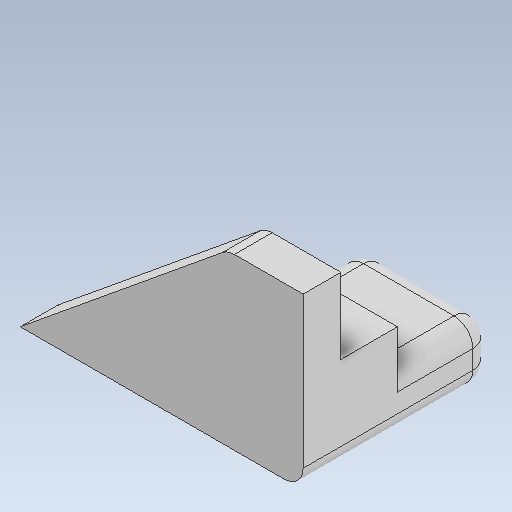
# Autodesk Inventor part: разделитель
Saved by Autodesk Inventor 2020 (Build 240168000, 168)
## iProperties
Created: 2022-07-30
Part Number: разделитель
Material: Типовые
Document SubType Name: Modeling
Designer: akapu
Density: 1 g/cm^3
Appearance: По умолчанию
Author: akapu
Autodesk Inventor part; units mm, degrees
ref_plane "YZ Plane" through (0, 0, 0) normal (1, 0, 0) x (0, 1, 0)
ref_plane "XZ Plane" through (0, 0, 0) normal (0, 1, 0) x (-1, 0, 0)
ref_plane "XY Plane" through (0, 0, 0) normal (0, 0, 1) x (1, 0, 0)
sketch "Эскиз1" plane through (0, 0, 0) normal (0, 0, 1) x (1, 0, 0)
  line L0 (0, 0) -> (0, 5)
  line L1 (0, 0) -> (-7, 0)
  line L2 (-7, 0) -> (0, 5)
  line L3 (0, 5) -> (4, 5)
  line L4 (4, 5) -> (4, 0)
  line L5 (4, 0) -> (0, 0)
  dimension "d0" = 5
  dimension "d1" = 7
  dimension "d2" = 4
  constraints: 12 end point, 2 perpendicular, 1 horizontal, 1 parallel, 1 point on line, 1 vertical
  measures "d0" distance of L0.start L0.end
  measures "d1" distance of L0.start L1.end
  measures "d2" distance of L0.end L3.end
extrude "Выдавливание1" add sketch "Эскиз1" along normal blind 3
sketch "Эскиз2" plane through (0, 0, 3) normal (0, 0, 1) x (1, 0, 0)
  line L0 (-7, 0) -> (4, 0) projected
  line L1 (-7, 0) -> (-11, 0)
  line L2 (4, 5) -> (0, 5) projected
  line L3 (0, 5) -> (0, 9)
  line L4 (0, 9) -> (-11, 0)
  line L5 (4, 5) -> (4, 9)
  line L6 (4, 9) -> (0, 9)
  line L7 (4, 0) -> (4, 5) projected
  line L8 (4, 5) -> (4, 0)
  line L9 (4, 0) -> (-7, 0)
  point P0 (0, 0)
  dimension "d5" = 4
  dimension "d6" = 4
  constraints: 14 end point, 2 collinear, 2 vertical, 1 horizontal, 1 perpendicular
  measures "d5" distance of L0.start L1.end
  measures "d6" distance of L2.end L3.end
extrude "Выдавливание2" add sketch "Эскиз2" along normal blind 2
sketch "Эскиз3" plane through (0, 0, 0) normal (0, 0, -1) x (-1, 0, 0)
  line L0 (-4, 0) -> (-4, 5) projected
  line L1 (-4, 0) -> (-4, 3)
  line L2 (-4, 3) -> (2.8, 3)
  line L3 (0, 5) -> (7, 0) projected
  line L4 (7, 0) -> (-4, 0) projected
  line L5 (2.8, 3) -> (7, 0)
  line L6 (7, 0) -> (-4, 0)
  line L7 (2.8, 3) -> (2.8, 0)
  point P0 (0, 0)
  dimension "d9" = 3
  constraints: 10 end point, 3 point on line, 2 perpendicular, 1 collinear
  measures "d9" distance of L0.start L1.end
extrude "Выдавливание3" add sketch "Эскиз3" along normal blind 5 contours L0 L2 L7 L4
fillet "Сопряжение1" radius 1 10 edges at (4, 3, -2.5) (4, 0, 0) (-2.8, 0, -2.5) (-2.8, 3, -2.5) (0, 5, 1.5) (0, 9, 4) (0.6, 3, -5) (4, 1.5, -5) (0.6, 0, -5) (-2.8, 1.5, -5)
